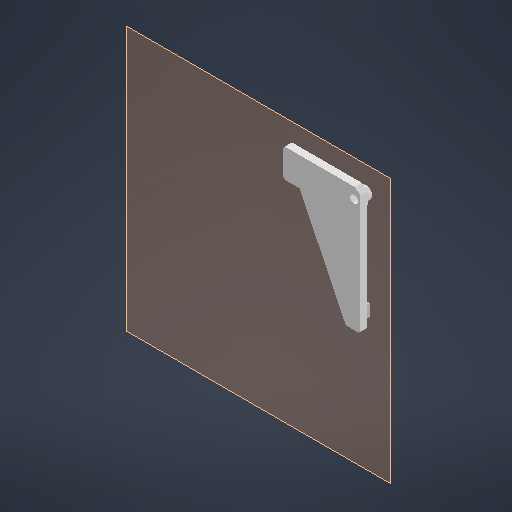
# Autodesk Inventor part: SnapHolder
Saved by Autodesk Inventor 2026.1 (Build 301233020, 233B)
## iProperties
Created: 2026-04-22
Part Number: SnapHolder
Material: Generic
Document SubType Name: Modeling
Designer: Mikke
Density: 1 g/cm^3
Appearance: Default
Author: Mikke
Autodesk Inventor part; units mm, degrees
ref_plane "YZ Plane" through (0, 0, 0) normal (1, 0, 0) x (0, 1, 0)
ref_plane "XZ Plane" through (0, 0, 0) normal (0, 1, 0) x (-1, 0, 0)
ref_plane "XY Plane" through (0, 0, 0) normal (0, 0, 1) x (1, 0, 0)
ref_plane "Work Plane1" through (0, 0, 0) normal (0, 0, 1) x (1, 0, 0)
sketch "Sketch1" plane through (0, 0, 0) normal (0, 0, 1) x (1, 0, 0)
  line L0 (104.1946, -29.0122) -> (104.1946, -34.0122) projected
  line L1 (107.1946, -29.0122) -> (104.1946, -29.0122) projected
  line L2 (107.1946, -34.0122) -> (107.1946, -29.0122) projected
  line L3 (104.1946, -34.0122) -> (107.1946, -34.0122) projected
  line L4 (126.4446, -68.7622) -> (123.4446, -68.7622) projected
  line L5 (123.4446, -68.7622) -> (123.4446, -73.7622) projected
  line L6 (126.4446, -73.7622) -> (126.4446, -68.7622) projected
  line L7 (123.4446, -73.7622) -> (126.4446, -73.7622) projected
  point P0 (0, 0)
extrude "Extrusion1" add sketch "Sketch1" along normal blind 2
sketch "Sketch2" plane through (126.4446, -73.7622, 0) normal (1, 0, 0) x (0, 0, -1)
  line L0 (0, 0) -> (0, 5) projected
  line L1 (0, 5) -> (-2, 5) projected
  line L2 (-2, 0) -> (-2, 5) projected
  line L3 (0, 0) -> (-2, 0) projected
  point P0 (0, 73.7622)
extrude "Extrusion2" cut sketch "Sketch2" against normal blind 1
sketch "Sketch3" plane through (107.1946, -34.0122, 0) normal (1, 0, 0) x (0, 0, -1)
  line L0 (0, 0) -> (0, 5) projected
  line L1 (0, 5) -> (-2, 5) projected
  line L2 (-2, 0) -> (-2, 5) projected
  line L3 (0, 0) -> (-2, 0) projected
  point P0 (0, 34.0122)
extrude "Extrusion3" cut sketch "Sketch3" against normal blind 1
sketch "Sketch4" plane through (0, 0, 0) normal (0, 0, -1) x (-1, 0, 0)
  line L0 (-125.4446, -68.7622) -> (-125.4446, -73.7622) projected
  line L1 (-123.4446, -73.7622) -> (-125.4446, -73.7622) projected
  line L2 (-123.4446, -68.7622) -> (-123.4446, -73.7622) projected
  line L3 (-125.4446, -68.7622) -> (-123.4446, -68.7622) projected
  line L4 (-106.1946, -29.0122) -> (-106.1946, -34.0122) projected
  line L5 (-104.1946, -34.0122) -> (-106.1946, -34.0122) projected
  line L6 (-104.1946, -29.0122) -> (-104.1946, -34.0122) projected
  line L7 (-106.1946, -29.0122) -> (-104.1946, -29.0122) projected
  point P0 (0, 0)
extrude "Extrusion4" add sketch "Sketch4" along normal blind 3.1
sketch "Sketch5" plane through (123.4446, -73.7622, 2) normal (-1, 0, 0) x (0, 0, 1)
  line L0 (-5.1558, 5) -> (-5.1558, 0) projected
  line L1 (-5.1, 0) -> (-5.1, 5) projected
  line L2 (0, 5) -> (-5.1, 5) projected
  line L3 (-5.1, 0) -> (0, 0) projected
  line L4 (-3.5558, 5) -> (-3.5558, 0) projected
  point P0 (-2, 73.7622)
extrude "Extrusion5" add sketch "Sketch5" along normal blind 0.9
sketch "Sketch6" plane through (104.1946, -34.0122, 2) normal (-1, 0, 0) x (0, 0, 1)
  line L0 (-5.1558, 5) -> (-5.1558, 0) projected
  line L1 (-5.1, 0) -> (-5.1, 5) projected
  line L2 (0, 0) -> (-5.1, 0) projected
  line L3 (-5.1, 5) -> (0, 5) projected
  line L4 (-5.1558, 5) -> (-5.1558, 0) projected
  line L5 (-3.5558, 5) -> (-3.5558, 0) projected
  point P0 (-2, 34.0122)
extrude "Extrusion6" add sketch "Sketch6" along normal blind 0.9
chamfer "Chamfer1" distance 1 angle 45 2 edges at (122.5446, -71.2622, -3.1) (103.2946, -31.5122, -3.1)
sketch "Sketch7" plane through (0, 0, 2) normal (0, 0, 1) x (1, 0, 0)
  line L0 (125.4446, -73.7622) -> (125.4446, -68.7622) projected
  line L1 (125.4446, -68.7622) -> (123.4446, -68.7622) projected
  line L2 (123.4446, -68.7622) -> (123.4446, -73.7622) projected
  line L3 (123.4446, -73.7622) -> (125.4446, -73.7622) projected
  line L4 (106.1946, -34.0122) -> (106.1946, -29.0122) projected
  line L5 (106.1946, -29.0122) -> (104.1946, -29.0122) projected
  line L6 (104.1946, -29.0122) -> (104.1946, -34.0122) projected
  line L7 (104.1946, -34.0122) -> (106.1946, -34.0122) projected
  line L8 (123.4446, -73.7622) -> (104.1946, -34.0122)
  line L9 (125.4446, -73.7622) -> (129.4446, -73.7622)
  line L10 (129.4446, -73.7622) -> (129.4446, -23.7622)
  line L11 (129.4446, -23.7622) -> (127.1946, -22.0122)
  line L12 (127.1946, -22.0122) -> (104.1946, -22.0122)
  line L13 (104.1946, -22.0122) -> (104.1946, -29.0122)
  circle A0 centre (126.8952, -26.4793) radius 1.25 projected
  circle A1 centre (126.8952, -26.4793) radius 1.65
  point P0 (0, 0)
  dimension "d15" = 4
  dimension "d16" = 50
  dimension "d17" = 7
  dimension "d18" = 23
  dimension "d21" = 0.4
  constraints: 12 end point, 1 centre point, 1 collinear, 1 horizontal, 1 parallel, 1 perpendicular
  measures "d15" distance of L0.start L9.end
  measures "d16" distance of L9.end L10.end
  measures "d17" distance of L12.end L5.end
  measures "d18" distance of L11.end L12.end
  measures "d21" radial gap between concentric circles of A0 A1
extrude "Extrusion7" add sketch "Sketch7" along normal blind 3 contours L3 L2 L1 L0 | L0 L1 L2 L8 L7 L4 L5 L13 L12 L11 L10 L9 | L6 L5 L4 L7
sketch "Sketch8" plane through (0, 0, 2) normal (0, 0, -1) x (-1, 0, 0)
  circle A0 centre (-126.8952, -26.4793) radius 1.65 projected
  circle A1 centre (-126.8952, -26.4793) radius 2.5529
  point P0 (0, 0)
  constraints: 1 centre point
extrude "Extrusion8" add sketch "Sketch8" along normal blind 2
fillet "Fillet1" radius 1 8 edges at (123.4446, -71.2622, 2) (125.4446, -71.2622, 2) (105.1946, -34.0122, 2) (106.1946, -31.5122, 2) (105.1946, -29.0122, 2) (126.8283, -23.9273, 2) (126.8283, -29.0314, 2) (124.4446, -68.7622, 2)
fillet "Fillet2" radius 1 3 edges at (129.4446, -73.7622, 3.5) (129.4446, -23.7622, 3.5) (127.1946, -22.0122, 3.5)
sketch "Sketch9" plane through (104.1946, -34.0122, -1.5558) normal (-1, 0, 0) x (0, 0, 1)
  line L0 (0, 5) -> (0, 0) projected
  line L1 (2.5558, 0) -> (0, 0) projected
  line L2 (6.5558, 0) -> (2.5558, 0) projected
  line L3 (6.5558, 12) -> (6.5558, 0) projected
  line L4 (3.5558, 12) -> (6.5558, 12) projected
  line L5 (3.5558, 12) -> (3.5558, 6) projected
  arc A0 (2.5558, 5) -> (3.5558, 6) centre (2.5558, 6) ccw projected
  line L6 (0, 5) -> (2.5558, 5) projected
  line L7 (6.5558, 0) -> (2.5558, 0) projected
  line L8 (6.5558, 12) -> (3.5558, 12)
  line L9 (3.5558, 12) -> (3.5558, 0)
  line L10 (3.5558, 0) -> (6.5558, 0)
  line L11 (6.5558, 0) -> (6.5558, 12)
  point P0 (1.5558, 34.0122)
  constraints: 8 end point, 2 parallel, 1 horizontal, 1 perpendicular, 1 point on line
extrude "Extrusion9" add sketch "Sketch9" along normal blind 6.7625 contours L5 L4 L3 L2 L9
fillet "Fillet3" radius 1 3 edges at (104.1946, -31.0122, 2) (97.4321, -34.0122, 3.5) (97.4321, -22.0122, 3.5)
body "Solid1"
